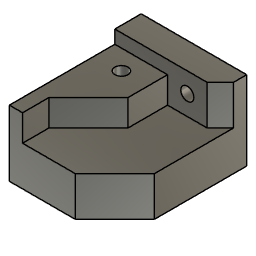
Task1a_2024A4PS0441P v1 (Autodesk Fusion 360 design; units mm, degrees)
Autodesk Fusion 360 part; units mm, degrees
sketch "Sketch1" plane through (0, 0, 0) normal (0, 0, 1) x (1, 0, 0)
  line L0 (0, 0) -> (50, 0)
  line L1 (0, 0) -> (0, 100)
  line L2 (0, 100) -> (80, 100)
  line L3 (80, 100) -> (80, 90)
  line L4 (80, 90) -> (80, 30)
  line L5 (50, 0) -> (80, 30)
  line L6 (0, 0) -> (10, 0)
  line L7 (10, 0) -> (10, 20)
  line L8 (0, 100) -> (0, 80)
  line L9 (0, 80) -> (70, 80)
  line L10 (70, 80) -> (80, 90)
  line L11 (0, 80) -> (40, 80)
  line L12 (40, 80) -> (40, 50)
  line L13 (10, 20) -> (40, 50)
  circle A0 centre (20, 65) radius 5
  constraint coincident L0.start L1.start
  constraint horizontal L0
  constraint perpendicular L0 L1
  constraint perpendicular L1 L2
  constraint perpendicular L2 L3
  constraint vertical L4
  constraint perpendicular L1 L6
  constraint perpendicular L6 L7
  constraint perpendicular L2 L8
  constraint perpendicular L1 L9
  constraint perpendicular L1 L11
  constraint perpendicular L9 L12
extrude "Extrude1" add sketch "Sketch1" along normal blind 50 contours L0 L1 L6 L7 L9 L11 L12 L13
extrude "Extrude2" add sketch "Sketch1" along normal blind 30 contours L0 L4 L5 L7 L9 L10 L12 L13
extrude "Extrude3" add sketch "Sketch1" along normal blind 60 contours L1 L2 L3 L8 L9 L10 L11
sketch "Sketch2" plane through (0, 80, 0) normal (0, -1, 0) x (1, 0, 0)
  line L0 (40, 30) -> (70, 30)
  line L1 (70, 30) -> (70, 60)
  line L2 (70, 60) -> (0, 60)
  line L3 (0, 60) -> (0, 50)
  line L4 (0, 50) -> (40, 50)
  line L5 (40, 50) -> (40, 30)
  circle A0 centre (55, 45) radius 5
extrude "Extrude4" cut sketch "Sketch2" against normal blind 40 contours A0
